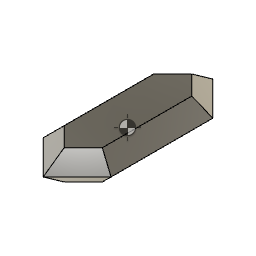
Rupee v2 (Autodesk Fusion 360 design; units mm, degrees)
Autodesk Fusion 360 part; units mm, degrees
sketch "Sketch1" plane through (0, 0, 0) normal (0, 0, 1) x (1, 0, 0)
  line L0 (0, 50) -> (-20, 30)
  line L1 (-20, 30) -> (-20, 0)
  line L2 (-20, 0) -> (-20, -30)
  line L3 (-20, -30) -> (0, -50)
  line L4 (0, -50) -> (20, -30)
  line L5 (20, -30) -> (20, 30)
  line L6 (20, 30) -> (0, 50)
  constraint vertical L1
  constraint parallel L1 L2
  constraint perpendicular L3 L4
  constraint parallel L2 L5
  constraint perpendicular L0 L6
extrude "Extrude1" add sketch "Sketch1" along normal blind 30
form "Form1" [no effect]
scale "Scale1" factor 2 about (20, -30, 30) bodies 1
extrude "Extrude2" cut 1 faces at (-6.6667, 30, 30) along direction (0, 0, -1) blind 25
move_body "Move1" bodies 1 to x (1, 0, 0) y (0, 1, 0) z (0, 0, 1) at (0, 0, 55)
move_body "Move2" bodies 1 to x (1, 0, 0) y (0, 1, 0) z (0, 0, 1) at (0, 0, -20)
chamfer "Chamfer1" distance 17.5 angle 45 1 edges at (20, 30, 40)
chamfer "Chamfer2" distance 17.5 angle 45 1 edges at (20, 30, 5)
chamfer "Chamfer3" distance 17.5 angle 45 1 edges at (-8.75, -58.75, 5)
chamfer "Chamfer4" distance 17.5 angle 45 1 edges at (-8.75, -58.75, 40)
chamfer "Chamfer5" distance 17.5 angle 45 1 edges at (-46.1872, -43.8128, 40)
chamfer "Chamfer6" distance 17.5 angle 45 1 edges at (-46.1872, -43.8128, 5)
chamfer "Chamfer7" distance 17.5 angle 45 1 edges at (-60, 42.3744, 40)
chamfer "Chamfer8" distance 17.5 angle 45 1 edges at (-60, 42.3744, 5)
chamfer "Chamfer9" distance 17.5 angle 45 1 edges at (-31.25, 118.75, 40)
chamfer "Chamfer10" distance 17.5 angle 45 1 edges at (-31.25, 118.75, 5)
chamfer "Chamfer11" distance 17.5 angle 45 1 edges at (-2.5628, 112.5628, 5)
chamfer "Chamfer12" distance 17.5 angle 45 1 edges at (-2.5628, 112.5628, 40)
scale "Scale2" factor 0.75 about (-42.5, 82.7513, 40) bodies 1
